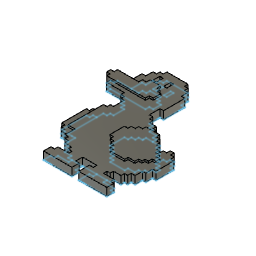
duck (Autodesk Fusion 360 design; units mm, degrees)
Autodesk Fusion 360 part; units mm, degrees
sketch "duck" plane through (0, 0, 0) normal (0, 0, 1) x (1, 0, 0)
  line L0 (27.4909, 0.0763) -> (27.4909, -9)
  line L1 (27.4909, -9) -> (25.6897, -9)
  line L2 (25.6897, -9) -> (25.6897, -12.5)
  line L3 (25.6897, -12.5) -> (24, -12.5)
  line L4 (24, -12.5) -> (24, -16.3541)
  line L5 (24, -16.3541) -> (22, -16.3541)
  line L6 (22, -16.3541) -> (22, -18.19)
  line L7 (22, -18.19) -> (20.3349, -18.19)
  line L8 (20.3349, -18.19) -> (20.3349, -20)
  line L9 (20.3349, -20) -> (16.5, -20)
  line L10 (16.5, -20) -> (16.5, -21.728)
  line L11 (16.5, -21.728) -> (14.8271, -21.728)
  line L12 (14.8271, -21.728) -> (14.8271, -23.5)
  line L13 (14.8271, -23.5) -> (20.3349, -23.5)
  line L14 (20.3349, -23.5) -> (20.3349, -25.2852)
  line L15 (20.3349, -25.2852) -> (22, -25.2852)
  line L16 (22, -25.2852) -> (22, -29)
  line L17 (22, -29) -> (7.5, -29)
  line L18 (7.5, -29) -> (7.5, -23.5)
  line L19 (7.5, -23.5) -> (9.5, -23.5)
  line L20 (9.5, -23.5) -> (9.5, -21.6707)
  line L21 (9.5, -21.6707) -> (2.1476, -21.6707)
  line L22 (2.1476, -21.6707) -> (2.1476, -25.2278)
  line L23 (2.1476, -25.2278) -> (4, -25.2278)
  line L24 (4, -25.2278) -> (4, -29)
  line L25 (4, -29) -> (-10.6517, -29)
  line L26 (-10.6517, -29) -> (-10.6517, -25.2278)
  line L27 (-10.6517, -25.2278) -> (-8.7502, -25.2278)
  line L28 (-8.7502, -25.2278) -> (-8.7502, -23.4492)
  line L29 (-8.7502, -23.4492) -> (-3.2062, -23.4492)
  line L30 (-3.2062, -23.4492) -> (-3.2062, -21.7434)
  line L31 (-3.2062, -21.7434) -> (-5.2451, -21.7434)
  line L32 (-5.2451, -21.7434) -> (-5.2451, -20)
  line L33 (-5.2451, -20) -> (-8.7502, -20)
  line L34 (-8.7502, -20) -> (-8.7502, -18)
  line L35 (-8.7502, -18) -> (-10.5829, -18)
  line L36 (-10.5829, -18) -> (-10.5829, -16.2452)
  line L37 (-10.5829, -16.2452) -> (-12.324, -16.2452)
  line L38 (-12.324, -16.2452) -> (-12.324, -14.5271)
  line L39 (-12.324, -14.5271) -> (-16, -14.5271)
  line L40 (-16, -14.5271) -> (-16, -12.6714)
  line L41 (-16, -12.6714) -> (-17.868, -12.6714)
  line L42 (-17.868, -12.6714) -> (-17.868, -10.7366)
  line L43 (-17.868, -10.7366) -> (-19.5, -10.7366)
  line L44 (-19.5, -10.7366) -> (-19.5, 2)
  line L45 (-19.5, 2) -> (-17.868, 2)
  line L46 (-17.868, 2) -> (-17.868, 3.7866)
  line L47 (-17.868, 3.7866) -> (-16, 3.7866)
  line L48 (-16, 3.7866) -> (-16, 7.2625)
  line L49 (-16, 7.2625) -> (-14.162, 7.2625)
  line L50 (-14.162, 7.2625) -> (-14.162, 9)
  line L51 (-14.162, 9) -> (-12.5, 9)
  line L52 (-12.5, 9) -> (-12.5, 14.5)
  line L53 (-12.5, 14.5) -> (-14.162, 14.5)
  line L54 (-14.162, 14.5) -> (-14.162, 16.2695)
  line L55 (-14.162, 16.2695) -> (-16, 16.2695)
  line L56 (-16, 16.2695) -> (-16, 18)
  line L57 (-16, 18) -> (-25.0921, 18)
  line L58 (-25.0921, 18) -> (-25.0921, 20)
  line L59 (-25.0921, 20) -> (-27, 20)
  line L60 (-27, 20) -> (-27, 21.6959)
  line L61 (-27, 21.6959) -> (-28.7391, 21.6959)
  line L62 (-28.7391, 21.6959) -> (-28.7391, 23.7396)
  line L63 (-28.7391, 23.7396) -> (-27, 23.7396)
  line L64 (-27, 23.7396) -> (-27, 25.5)
  line L65 (-27, 25.5) -> (-19.8067, 25.5)
  line L66 (-19.8067, 25.5) -> (-19.8067, 31)
  line L67 (-19.8067, 31) -> (-17.851, 31)
  line L68 (-17.851, 31) -> (-17.851, 34.6981)
  line L69 (-17.851, 34.6981) -> (-16, 34.6981)
  line L70 (-16, 34.6981) -> (-16, 36.4071)
  line L71 (-16, 36.4071) -> (-14.1865, 36.4071)
  line L72 (-14.1865, 36.4071) -> (-14.1865, 38.1865)
  line L73 (-14.1865, 38.1865) -> (-3.1927, 38.1865)
  line L74 (-3.1927, 38.1865) -> (-3.1927, 36.4071)
  line L75 (-3.1927, 36.4071) -> (-1.3428, 36.4071)
  line L76 (-1.3428, 36.4071) -> (-1.3428, 34.5)
  line L77 (-1.3428, 34.5) -> (0.5, 34.5)
  line L78 (0.5, 34.5) -> (0.5, 31)
  line L79 (0.5, 31) -> (2.3218, 31)
  line L80 (2.3218, 31) -> (2.3218, 20)
  line L81 (2.3218, 20) -> (0.5, 20)
  line L82 (0.5, 20) -> (0.5, 14.5)
  line L83 (0.5, 14.5) -> (2.3218, 14.5)
  line L84 (2.3218, 14.5) -> (2.3218, 12.6948)
  line L85 (2.3218, 12.6948) -> (4.1193, 12.6948)
  line L86 (4.1193, 12.6948) -> (4.1193, 11)
  line L87 (4.1193, 11) -> (7.7144, 11)
  line L88 (7.7144, 11) -> (7.7144, 9.1465)
  line L89 (7.7144, 9.1465) -> (9.5, 9.1465)
  line L90 (9.5, 9.1465) -> (9.5, 7.2945)
  line L91 (9.5, 7.2945) -> (13.1302, 7.2945)
  line L92 (13.1302, 7.2945) -> (13.1302, 5.5)
  line L93 (13.1302, 5.5) -> (15, 5.5)
  line L94 (15, 5.5) -> (15, 3.7617)
  line L95 (15, 3.7617) -> (16.7253, 3.7617)
  line L96 (16.7253, 3.7617) -> (16.7253, 2)
  line L97 (16.7253, 2) -> (18.5, 2)
  line L98 (18.5, 2) -> (18.5, 0.1356)
  line L99 (18.5, 0.1356) -> (20.1958, 0.1356)
  line L100 (20.1958, 0.1356) -> (20.1958, 2)
  line L101 (20.1958, 2) -> (22, 2)
  line L102 (22, 2) -> (22, 3.824)
  line L103 (22, 3.824) -> (24, 3.824)
  line L104 (24, 3.824) -> (24, 2)
  line L105 (24, 2) -> (25.814, 2)
  line L106 (25.814, 2) -> (25.814, 0.0763)
  line L107 (25.814, 0.0763) -> (27.4909, 0.0763)
  line L108 (-19.8067, 25.5) -> (-16, 25.5)
  line L109 (-16, 25.5) -> (-16, 27.4565)
  line L110 (-16, 27.4565) -> (-14, 27.4565)
  line L111 (-14, 27.4565) -> (-14, 29.3547)
  line L112 (-14, 29.3547) -> (-8.5527, 29.3547)
  line L113 (-8.5527, 29.3547) -> (-8.5527, 27.4565)
  line L114 (-8.5527, 27.4565) -> (-7, 27.4565)
  line L115 (-7, 27.4565) -> (-7, 26)
  line L116 (-7, 26) -> (-5, 26)
  line L117 (-5, 26) -> (-5, 22)
  line L118 (-5, 22) -> (-7, 22)
  line L119 (-7, 22) -> (-7, 20)
  line L120 (-7, 20) -> (-25.0921, 20)
  line L121 (-8.5, 34.5) -> (-7, 34.5)
  line L122 (-7, 34.5) -> (-7, 31)
  line L123 (-7, 31) -> (-8.5, 31)
  line L124 (-8.5, 31) -> (-8.5, 34.5)
  line L125 (-14.0411, 34.4298) -> (-12.2623, 34.4298)
  line L126 (-12.2623, 34.4298) -> (-12.2623, 31)
  line L127 (-12.2623, 31) -> (-14.0411, 31)
  line L128 (-14.0411, 31) -> (-14.0411, 34.4298)
  line L129 (-16, 3.7866) -> (-16, -11)
  line L130 (-16, -11) -> (-14, -11)
  line L131 (-14, -11) -> (-12.324, -11)
  line L132 (-12.324, -11) -> (-12.324, -14.5271)
  line L133 (-3.2062, -21.7434) -> (2.1476, -21.6707)
  line L134 (9.5, -21.6707) -> (14.8271, -21.728)
  line L135 (9.5, 7.2945) -> (6, 7.2945)
  line L136 (6, 7.2945) -> (6, 6)
  line L137 (6, 6) -> (6, 5.5)
  line L138 (6, 5.5) -> (4, 5.5)
  line L139 (4, 5.5) -> (4, 3.7432)
  line L140 (4, 3.7432) -> (2, 3.7432)
  line L141 (2, 3.7432) -> (2, 2)
  line L142 (2, 2) -> (0.1455, 2)
  line L143 (0.1455, 2) -> (0.1455, -5.5)
  line L144 (0.1455, -5.5) -> (2, -5.5)
  line L145 (2, -5.5) -> (2, -7.263)
  line L146 (2, -7.263) -> (4, -7.263)
  line L147 (4, -7.263) -> (4, -9)
  line L148 (4, -9) -> (5.7483, -9)
  line L149 (5.7483, -9) -> (5.7483, -11)
  line L150 (5.7483, -11) -> (7.5, -11)
  line L151 (7.5, -11) -> (7.5, -12.7164)
  line L152 (7.5, -12.7164) -> (15, -12.7164)
  line L153 (15, -12.7164) -> (15, -11)
  line L154 (15, -11) -> (18.5, -11)
  line L155 (18.5, -11) -> (18.5, -9)
  line L156 (18.5, -9) -> (20.2656, -9)
  line L157 (20.2656, -9) -> (20.2656, -7.5)
  line L158 (20.2656, -7.5) -> (22, -7.5)
  line L159 (22, -7.5) -> (22, -5.5)
  line L160 (22, -5.5) -> (24, -5.5)
  line L161 (24, -5.5) -> (24, -3.5)
  line L162 (24, -3.5) -> (22, -3.5)
  line L163 (22, -3.5) -> (22, -1.7101)
  line L164 (22, -1.7101) -> (20, -1.7101)
  line L165 (20, -1.7101) -> (20, 0.1356)
  constraint vertical L0
  constraint perpendicular L0 L1
  constraint perpendicular L1 L2
  constraint perpendicular L0 L3
  constraint perpendicular L3 L4
  constraint perpendicular L4 L5
  constraint perpendicular L5 L6
  constraint perpendicular L6 L7
  constraint perpendicular L7 L8
  constraint perpendicular L8 L9
  constraint perpendicular L7 L10
  constraint perpendicular L8 L11
  constraint perpendicular L11 L12
  constraint perpendicular L12 L13
  constraint perpendicular L11 L14
  constraint perpendicular L12 L15
  constraint perpendicular L11 L16
  constraint perpendicular L16 L17
  constraint perpendicular L11 L18
  constraint perpendicular L18 L19
  constraint perpendicular L19 L20
  constraint perpendicular L18 L21
  constraint perpendicular L21 L22
  constraint perpendicular L22 L23
  constraint perpendicular L23 L24
  constraint perpendicular L24 L25
  constraint perpendicular L25 L26
  constraint perpendicular L24 L27
  constraint perpendicular L27 L28
  constraint perpendicular L24 L29
  constraint perpendicular L27 L30
  constraint perpendicular L24 L31
  constraint perpendicular L27 L32
  constraint perpendicular L24 L33
  constraint perpendicular L33 L34
  constraint perpendicular L34 L35
  constraint perpendicular L35 L36
  constraint perpendicular L36 L37
  constraint perpendicular L37 L38
  constraint perpendicular L38 L39
  constraint perpendicular L39 L40
  constraint perpendicular L40 L41
  constraint perpendicular L41 L42
  constraint perpendicular L40 L43
  constraint perpendicular L41 L44
  constraint perpendicular L44 L45
  constraint perpendicular L39 L46
  constraint perpendicular L44 L47
  constraint perpendicular L47 L48
  constraint perpendicular L44 L49
  constraint perpendicular L49 L50
  constraint perpendicular L44 L51
  constraint perpendicular L51 L52
  constraint perpendicular L52 L53
  constraint perpendicular L51 L54
  constraint perpendicular L54 L55
  constraint perpendicular L51 L56
  constraint perpendicular L52 L57
  constraint perpendicular L57 L58
  constraint perpendicular L58 L59
  constraint perpendicular L57 L60
  constraint perpendicular L58 L61
  constraint perpendicular L57 L62
  constraint perpendicular L58 L63
  constraint perpendicular L63 L64
  constraint perpendicular L58 L65
  constraint perpendicular L65 L66
  constraint perpendicular L66 L67
  constraint perpendicular L65 L68
  constraint perpendicular L68 L69
  constraint perpendicular L69 L70
  constraint perpendicular L68 L71
  constraint perpendicular L71 L72
  constraint perpendicular L72 L73
  constraint perpendicular L73 L74
  constraint perpendicular L74 L75
  constraint perpendicular L73 L76
  constraint perpendicular L74 L77
  constraint perpendicular L77 L78
  constraint perpendicular L74 L79
  constraint perpendicular L79 L80
  constraint perpendicular L80 L81
  constraint perpendicular L81 L82
  constraint perpendicular L82 L83
  constraint perpendicular L83 L84
  constraint perpendicular L82 L85
  constraint perpendicular L83 L86
  constraint perpendicular L82 L87
  constraint perpendicular L87 L88
  constraint perpendicular L82 L89
  constraint perpendicular L89 L90
  constraint perpendicular L90 L91
  constraint perpendicular L89 L92
  constraint perpendicular L92 L93
  constraint perpendicular L93 L94
  constraint perpendicular L92 L95
  constraint perpendicular L95 L96
  constraint perpendicular L96 L97
  constraint perpendicular L95 L98
  constraint perpendicular L96 L99
  constraint perpendicular L99 L100
  constraint perpendicular L100 L101
  constraint perpendicular L99 L102
  constraint perpendicular L100 L103
  constraint perpendicular L99 L104
  constraint perpendicular L104 L105
  constraint perpendicular L99 L106
  constraint perpendicular L106 L107
  constraint perpendicular L66 L108
  constraint perpendicular L65 L109
  constraint perpendicular L109 L110
  constraint perpendicular L65 L111
  constraint perpendicular L111 L112
  constraint perpendicular L112 L113
  constraint perpendicular L113 L114
  constraint perpendicular L114 L115
  constraint perpendicular L113 L116
  constraint perpendicular L114 L117
  constraint perpendicular L117 L118
  constraint perpendicular L114 L119
  constraint perpendicular L117 L120
  constraint horizontal L121
  constraint perpendicular L121 L122
  constraint perpendicular L122 L123
  constraint perpendicular L123 L124
  constraint horizontal L125
  constraint perpendicular L125 L126
  constraint perpendicular L126 L127
  constraint perpendicular L125 L128
  constraint perpendicular L47 L129
  constraint perpendicular L129 L130
  constraint perpendicular L129 L131
  constraint perpendicular L131 L132
  constraint perpendicular L90 L135
  constraint perpendicular L91 L136
  constraint perpendicular L91 L137
  constraint perpendicular L136 L138
  constraint perpendicular L91 L139
  constraint perpendicular L136 L140
  constraint perpendicular L140 L141
  constraint perpendicular L136 L142
  constraint perpendicular L140 L143
  constraint perpendicular L143 L144
  constraint perpendicular L144 L145
  constraint perpendicular L143 L146
  constraint perpendicular L146 L147
  constraint perpendicular L147 L148
  constraint perpendicular L146 L149
  constraint perpendicular L147 L150
  constraint perpendicular L150 L151
  constraint perpendicular L147 L152
  constraint perpendicular L150 L153
  constraint perpendicular L153 L154
  constraint perpendicular L154 L155
  constraint perpendicular L155 L156
  constraint perpendicular L154 L157
  constraint perpendicular L155 L158
  constraint perpendicular L154 L159
  constraint perpendicular L159 L160
  constraint perpendicular L154 L161
  constraint perpendicular L159 L162
  constraint perpendicular L162 L163
  constraint perpendicular L159 L164
  constraint coincident L99 L165.end
  constraint perpendicular L99 L165
extrude "Extrude1" add sketch "duck" along normal blind 4 contours L0 L1 L2 L3 L4 L5 L6 L7 L8 L9 L10 L11 L21 L31 L32 L33 L34 L35 L36 L37 L38 L48 L49 L50 L51 L52 L53 L54 L55 L56 L57 L58 L66 L67 L68 L69 L70 L71 L72 L73 L74 L75 L76 L77 L78 L79 L80 L81 L82 L83 L84 L85 L86 L87 L88 L89 L90 L99 L100 L101 L102 L103 L104 L105 L106 L107 L108 L109 L110 L111 L112 L113 L114 L115 L116 L117 L118 L119 L120 L129 L130 L131 L132 L133 L134 L135 L136 L137 L138 L139 L140 L141 L142 L143 L144 L145 L146 L147 L148 L149 L150 L151 L152 L153 L154 L155 L156 L157 L158 L159 L160 L161 L162 L163 L164 L165 | L12 L13 L14 L15 L16 L17 L18 L19 L20 L134 | L22 L23 L24 L25 L26 L27 L28 L29 L30 L133
extrude "Extrude2" add sketch "duck" along normal blind 5 contours L91 L92 L93 L94 L95 L96 L97 L98 L99 L135 L136 L137 L138 L139 L140 L141 L142 L143 L144 L145 L146 L147 L148 L149 L150 L151 L152 L153 L154 L155 L156 L157 L158 L159 L160 L161 L162 L163 L164 L165
extrude "Extrude3" add sketch "duck" along normal blind 5 contours L59 L60 L61 L62 L63 L64 L65 L108 L109 L110 L111 L112 L113 L114 L115 L116 L117 L118 L119 L120
extrude "Extrude4" add sketch "duck" along normal blind 3 contours L39 L40 L41 L42 L43 L44 L45 L46 L47 L129 L130 L131 L132
named bodies: "duck"
